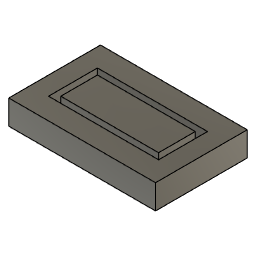
Day #14 Slot Box v1 (Autodesk Fusion 360 design; units mm, degrees)
Autodesk Fusion 360 part; units mm, degrees
sketch "Sketch1" plane through (0, 0, 0) normal (0, 0, 1) x (1, 0, 0)
  line L0 (60, 37.5) -> (-60, 37.5)
  line L1 (-60, 37.5) -> (-60, -37.5)
  line L2 (-60, -37.5) -> (60, -37.5)
  line L3 (60, -37.5) -> (60, 37.5)
  line L4 (60, 37.5) -> (-60, -37.5) construction
  line L5 (-60, 37.5) -> (60, -37.5) construction
  line L6 (45, 20) -> (-45, 20)
  line L7 (-45, 20) -> (-45, -20)
  line L8 (-45, -20) -> (45, -20)
  line L9 (45, -20) -> (45, 20)
  line L10 (45, 20) -> (-45, -20) construction
  line L11 (-45, 20) -> (45, -20) construction
  line L12 (-40, 15) -> (40, 15)
  line L13 (40, 15) -> (40, -15)
  line L14 (40, -15) -> (-40, -15)
  line L15 (-40, -15) -> (-40, 15)
  line L16 (-40, 15) -> (40, -15) construction
  line L17 (40, 15) -> (-40, -15) construction
  dimension "d1" = 120
  dimension "d2" = 75
  dimension "d3" = 90
  dimension "d4" = 40
  dimension "d5" = 80
  dimension "d6" = 30
  constraint horizontal L0
  constraint perpendicular L0 L1
  constraint parallel L0 L2
  constraint parallel L1 L3
  constraint coincident L4 origin
  constraint coincident L5 origin
  constraint horizontal L6
  constraint perpendicular L6 L7
  constraint parallel L6 L8
  constraint parallel L7 L9
  constraint coincident L10 origin
  constraint coincident L11 origin
  constraint horizontal L12
  constraint perpendicular L12 L13
  constraint parallel L12 L14
  constraint parallel L13 L15
  constraint coincident L16 origin
  constraint coincident L17 origin
  measures "d1" distance of L1.end L2.end
  measures "d2" distance of L0.end L1.end
  measures "d3" distance of L7.end L8.end
  measures "d4" distance of L6.end L7.end
  measures "d5" distance of L13.end L14.end
  measures "d6" distance of L12.end L13.end
extrude "Extrude1" add sketch "Sketch1" along normal blind 20 makes body 1 at (15, -31.6667, 0) makes body 2 at (-13.3333, -5, 0)
extrude "Extrude2" add sketch "Sketch1" along normal blind 5 contours L6 L7 L8 L9 bodies 1 2
